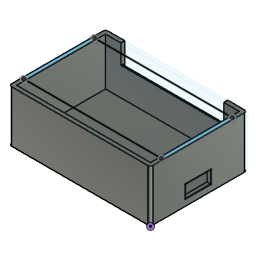
electronics-housing (Autodesk Fusion 360 design; units mm, degrees)
Autodesk Fusion 360 part; units mm, degrees
sketch "Sketch1" plane through (0, 0, 0) normal (0, 0, 1) x (1, 0, 0)
  line L0 (0, 0) -> (110, 0)
  line L1 (110, 0) -> (110, 75)
  line L2 (110, 75) -> (0, 75)
  line L3 (0, 75) -> (0, 0)
  dimension "d1" = 110
  dimension "d2" = 75
  constraint horizontal L0
  constraint vertical L1
  constraint horizontal L2
  constraint vertical L3
  constraint coincident L0.start L3.end
  measures "d1" distance of L0.start L0.end
  measures "d2" distance of L0.start L2.end
extrude "Extrude1" add sketch "Sketch1" along normal blind 40
shell "Shell1" thickness 3 removed faces 1 at (36.6667, 50, 40)
sketch "Sketch2" plane through (0, 0, 40) normal (0, 0, 1) x (-1, 0, 0)
  line L0 (-3, -72) -> (-107, -72)
  line L1 (-107, -72) -> (-107, -3)
  line L2 (-107, -3) -> (-3, -3)
  line L3 (-3, -3) -> (-3, -72)
  line L4 (0, -75) -> (0, 0)
  line L5 (0, 0) -> (-110, 0)
  line L6 (-110, 0) -> (-110, -75)
  line L7 (-110, -75) -> (0, -75)
  line L8 (-1.5, -10) -> (-108.5, -10)
  line L9 (-108.5, -10) -> (-108.5, -65)
  line L10 (-108.5, -65) -> (-1.5, -65)
  line L11 (-1.5, -65) -> (-1.5, -10)
  point P0 (-1.5, -65)
  point P1 (-108.5, -65)
  point P2 (-108.5, -10)
  point P3 (-1.5, -10)
  dimension "d31" = 10
  dimension "d32" = 65
  constraint horizontal L8
  constraint vertical L9
  constraint horizontal L10
  constraint vertical L11
  constraint coincident P0 L10.end
  constraint coincident P1 L9.end
  constraint coincident P2 L8.end
  constraint coincident P3 L8.start
  measures "d31" distance of L5 L8
  measures "d32" distance of L5 L10
hole "Hole1" at (1.5, 65, 40) at (108.5, 65, 40) at (108.5, 10, 40) at (1.5, 10, 40) direction (0, 0, -1) diameter 2 depth 3 tip angle 180
sketch "Sketch3" plane through (0, 75, 0) normal (0, 1, 0) x (-1, 0, 0)
  line L0 (-110, 0) -> (0, 0)
  line L1 (0, 0) -> (0, 40)
  line L2 (0, 40) -> (-110, 40)
  line L3 (-110, 40) -> (-110, 0)
  line L4 (-95, 45) -> (-15, 45)
  line L5 (-15, 45) -> (-15, 25)
  line L6 (-15, 25) -> (-95, 25)
  line L7 (-95, 25) -> (-95, 45)
  line L8 (-80, 39.9808) -> (-30, 39.9808)
  line L9 (-30, 39.9808) -> (-30, 45)
  line L10 (-30, 45) -> (-80, 45)
  line L11 (-80, 45) -> (-80, 39.9808)
  dimension "d22" = 15
  dimension "d25" = 80
  dimension "d26" = 15
  dimension "d27" = 50
  dimension "d28" = 20
  dimension "d33" = 25
  constraint horizontal L4
  constraint vertical L5
  constraint horizontal L6
  constraint vertical L7
  constraint horizontal L8
  constraint vertical L9
  constraint horizontal L10
  constraint vertical L11
  constraint coincident L4 L9.end
  measures "d22" horizontal distance of L0.end L5.end
  measures "d25" distance of L4.start L4.end
  measures "d26" distance of L5 L9
  measures "d27" distance of L8.start L8.end
  measures "d28" distance of L4 L6
  measures "d33" distance of L0.end L6
sketch "Sketch5" plane through (110, 0, 0) normal (1, 0, 0) x (0, 1, 0)
  line L0 (0, 0) -> (75, 0)
  line L1 (75, 0) -> (75, 40)
  line L2 (75, 40) -> (0, 40)
  line L3 (0, 40) -> (0, 0)
  line L4 (27, 5) -> (47, 5)
  line L5 (47, 5) -> (47, 15)
  line L6 (47, 15) -> (27, 15)
  line L7 (27, 15) -> (27, 5)
  dimension "d11" = 20
  dimension "d12" = 10
  dimension "d16" = 27
  dimension "d17" = 5
  constraint horizontal L4
  constraint vertical L5
  constraint horizontal L6
  constraint vertical L7
  measures "d11" distance of L4.start L4.end
  measures "d12" distance of L4.start L6.end
  measures "d16" horizontal distance of L0.start L4.start
  measures "d17" vertical distance of L0.end L4.end
extrude "Extrude3" cut sketch "Sketch5" against normal blind 5 contours L4 L5 L6 L7
extrude "Extrude4" cut sketch "Sketch3" against normal blind 5 contours L2 L4 L7 L11 | L2 L5 L6 L7 L8 | L2 L4 L5 L9 | L2 L4 L8 L9 L10 L11
fillet "Fillet1" radius 2 1 edges at (110, 75, 20)
fillet "Fillet2" radius 2 1 edges at (110, 0, 20)
fillet "Fillet2" radius 2 1 edges at (0, 0, 20)
fillet "Fillet2" radius 2 1 edges at (0, 75, 20)
fillet "Fillet2" radius 2 1 edges at (55, 75, 25)
equation "d22 = ( 110 / 2 ) * 1 mm - d25 / 2"
equation "d26 = d25 / 2 - d27 / 2"
equation "d32 = 75 mm - d31"
